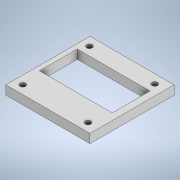
# Autodesk Inventor part: Test OLED
Saved by Autodesk Inventor 2021 (Build 250183000, 183)
## iProperties
Created: 2021-08-04
Part Number: Test OLED
Material: Generic
Document SubType Name: Modeling
Designer: cmzgt
Density: 1 g/cm^3
Appearance: Default
Author: cmzgt
Autodesk Inventor part; units mm, degrees
ref_plane "YZ Plane" through (0, 0, 0) normal (1, 0, 0) x (0, 1, 0)
ref_plane "XZ Plane" through (0, 0, 0) normal (0, 1, 0) x (-1, 0, 0)
ref_plane "XY Plane" through (0, 0, 0) normal (0, 0, 1) x (1, 0, 0)
sketch "Sketch3" plane through (0, 0, 0) normal (0, 1, 0) x (-1, 0, 0)
  line L0 (-15, -15) -> (15, -15)
  line L1 (15, -15) -> (15, 15)
  line L2 (15, 15) -> (-15, 15)
  line L3 (-15, 15) -> (-15, -15)
  line L4 (-15, -15) -> (15, 15) construction
  line L5 (15, -15) -> (-15, 15) construction
  point P0 (0, 0)
  dimension "d0" = 30
  dimension "d1" = 30
  constraints: 12 end point, 2 midpoint, 2 parallel, 1 horizontal, 1 perpendicular
  measures "d0" distance of L2.end L1.end
  measures "d1" distance of L1.end L0.end
extrude "Extrusion1" add sketch "Sketch3" along normal blind 3.2
sketch "Sketch5" plane through (0, 3.2, 0) normal (0, 1, 0) x (1, 0, 0)
  line L0 (-14, -14) -> (13.3, -14)
  line L1 (13.3, -14) -> (13.3, 13.8)
  line L2 (13.3, 13.8) -> (-14, 13.8)
  line L3 (-14, 13.8) -> (-14, -14)
  circle A0 centre (-12, 11.8) radius 1
  line L4 (-0.35, 13.8) -> (-0.35, -14) construction
  line L5 (-14, -0.1) -> (13.3, -0.1) construction
  circle A1 centre (11.3, 11.8) radius 1
  circle A2 centre (-12, -12) radius 1
  circle A3 centre (11.3, -12) radius 1
  line L6 (12.65, -4.7) -> (-13.35, -4.7)
  line L7 (-13.35, -4.7) -> (-13.35, 8.8)
  line L8 (-13.35, 8.8) -> (12.65, 8.8)
  line L9 (12.65, 8.8) -> (12.65, -4.7)
  line L10 (12.65, -4.7) -> (-13.35, 8.8) construction
  line L11 (-13.35, -4.7) -> (12.65, 8.8) construction
  line L12 (13, -9.73) -> (-13.7, -9.73)
  line L13 (-13.7, -9.73) -> (-13.7, 9.53)
  line L14 (-13.7, 9.53) -> (13, 9.53)
  line L15 (13, 9.53) -> (13, -9.73)
  line L16 (13, -9.73) -> (-13.7, 9.53) construction
  line L17 (-13.7, -9.73) -> (13, 9.53) construction
  line L18 (-15, -15) -> (15, -15) projected
  line L19 (-15, 15) -> (-15, -15) projected
  point P0 (44.7499, 0)
  point P1 (-0.35, 2.05)
  point P2 (-0.35, -0.1)
  dimension "d4" = 27.3
  dimension "d5" = 27.8
  dimension "d7" = 2
  dimension "d8" = 2
  dimension "d9" = 2
  dimension "d10" = 26
  dimension "d11" = 13.5
  dimension "d12" = 5
  dimension "d13" = 26.7
  dimension "d14" = 19.26
  dimension "d15" = 4.27
  dimension "d17" = 1
  dimension "d18" = 1
  constraints: 36 end point, 9 midpoint, 6 parallel, 4 centre point, 3 horizontal, 3 perpendicular, 3 symmetric about line, 1 point on line, 3 other
  measures "d4" distance of L2.end L1.end
  measures "d5" distance of L1.end L0.end
  measures "d7" diameter of A0
  measures "d8" distance from line of L2 A0.centre
  measures "d9" distance from line of L3 A0.centre
  measures "d10" distance of L7.end L8.end
  measures "d11" distance of L6.end L7.end
  measures "d12" distance between parallel lines of L2 L8
  measures "d13" distance of L13.end L14.end
  measures "d14" distance of L12.end L13.end
  measures "d15" distance between parallel lines of L2 L14
  measures "d17" distance between parallel lines of L18 L0
  measures "d18" distance between parallel lines of L19 L3
extrude "Extrusion2" cut sketch "Sketch5" against normal up to surface (3.2 mm away) contours A0 | A1 | A2 | A3 | L6 L7 L8 L9
body "Solid1"
